Autodesk Inventor part; units mm, degrees
(part 3 of 3)
  arc A48 (19.7098, 5.9019) -> (19.4526, 6.1717) centre (13.25, 0) ccw
  line L1883 (19.7098, 5.9019) -> (19.6582, 5.7672)
  line L1884 (19.6582, 5.7672) -> (19.6285, 5.6961)
  line L1885 (19.6285, 5.6961) -> (19.5685, 5.5641)
  line L1886 (19.5685, 5.5641) -> (19.5095, 5.4477)
  line L1887 (19.5095, 5.4477) -> (19.4525, 5.3459)
  line L1888 (19.4525, 5.3459) -> (19.3981, 5.2575)
  line L1889 (19.3981, 5.2575) -> (19.348, 5.1833)
  line L1890 (19.348, 5.1833) -> (19.3013, 5.1201)
  line L1891 (19.3013, 5.1201) -> (19.2635, 5.0732)
  line L1892 (19.2635, 5.0732) -> (19.2071, 5.0072)
  line L1893 (19.2071, 5.0072) -> (19.1891, 4.9822)
  line L1894 (19.1891, 4.9822) -> (19.1747, 4.9588)
  line L1895 (19.1747, 4.9588) -> (19.1639, 4.937)
  line L1896 (19.1639, 4.937) -> (19.1565, 4.917)
  line L1897 (19.1565, 4.917) -> (19.1525, 4.8989)
  line L1898 (19.1525, 4.8989) -> (19.1519, 4.8829)
  line L1899 (19.1519, 4.8829) -> (19.1544, 4.869)
  line L1900 (19.1544, 4.869) -> (19.1601, 4.8575)
  line L1901 (19.1601, 4.8575) -> (19.1753, 4.8388)
  line L1902 (19.1753, 4.8388) -> (19.2633, 4.7289)
  line L1903 (19.2633, 4.7289) -> (19.3493, 4.6175)
  line L1904 (19.3493, 4.6175) -> (19.3639, 4.5983)
  line L1905 (19.3639, 4.5983) -> (19.3738, 4.5901)
  line L1906 (19.3738, 4.5901) -> (19.3867, 4.5843)
  line L1907 (19.3867, 4.5843) -> (19.4024, 4.5812)
  line L1908 (19.4024, 4.5812) -> (19.4209, 4.5808)
  line L1909 (19.4209, 4.5808) -> (19.4421, 4.5832)
  line L1910 (19.4421, 4.5832) -> (19.4658, 4.5886)
  line L1911 (19.4658, 4.5886) -> (19.492, 4.5971)
  line L1912 (19.492, 4.5971) -> (19.5205, 4.6087)
  line L1913 (19.5205, 4.6087) -> (19.5979, 4.6479)
  line L1914 (19.5979, 4.6479) -> (19.6525, 4.6736)
  line L1915 (19.6525, 4.6736) -> (19.7249, 4.7041)
  line L1916 (19.7249, 4.7041) -> (19.8088, 4.7352)
  line L1917 (19.8088, 4.7352) -> (19.9076, 4.7673)
  line L1918 (19.9076, 4.7673) -> (20.0198, 4.7987)
  line L1919 (20.0198, 4.7987) -> (20.1469, 4.8286)
  line L1920 (20.1469, 4.8286) -> (20.2894, 4.8558)
  line L1921 (20.2894, 4.8558) -> (20.3654, 4.8679)
  line L1922 (20.3654, 4.8679) -> (20.5085, 4.8863)
  arc A49 (20.7101, 4.5727) -> (20.5085, 4.8863) centre (13.25, 0) ccw
  line L1923 (20.7101, 4.5727) -> (20.6338, 4.4502)
  line L1924 (20.6338, 4.4502) -> (20.5912, 4.3861)
  line L1925 (20.5912, 4.3861) -> (20.5073, 4.2678)
  line L1926 (20.5073, 4.2678) -> (20.4273, 4.1646)
  line L1927 (20.4273, 4.1646) -> (20.3522, 4.0755)
  line L1928 (20.3522, 4.0755) -> (20.2819, 3.999)
  line L1929 (20.2819, 3.999) -> (20.2187, 3.9356)
  line L1930 (20.2187, 3.9356) -> (20.1609, 3.8824)
  line L1931 (20.1609, 3.8824) -> (20.1149, 3.8434)
  line L1932 (20.1149, 3.8434) -> (20.0471, 3.7893)
  line L1933 (20.0471, 3.7893) -> (20.0247, 3.7682)
  line L1934 (20.0247, 3.7682) -> (20.0061, 3.7479)
  line L1935 (20.0061, 3.7479) -> (19.9914, 3.7286)
  line L1936 (19.9914, 3.7286) -> (19.9803, 3.7103)
  line L1937 (19.9803, 3.7103) -> (19.973, 3.6933)
  line L1938 (19.973, 3.6933) -> (19.9693, 3.6777)
  line L1939 (19.9693, 3.6777) -> (19.9692, 3.6636)
  line L1940 (19.9692, 3.6636) -> (19.9726, 3.6512)
  line L1941 (19.9726, 3.6512) -> (19.9839, 3.63)
  line L1942 (19.9839, 3.63) -> (20.0496, 3.5054)
  line L1943 (20.0496, 3.5054) -> (20.113, 3.3797)
  line L1944 (20.113, 3.3797) -> (20.1237, 3.3581)
  line L1945 (20.1237, 3.3581) -> (20.1318, 3.3482)
  line L1946 (20.1318, 3.3482) -> (20.1434, 3.3401)
  line L1947 (20.1434, 3.3401) -> (20.1582, 3.3341)
  line L1948 (20.1582, 3.3341) -> (20.1763, 3.3302)
  line L1949 (20.1763, 3.3302) -> (20.1976, 3.3286)
  line L1950 (20.1976, 3.3286) -> (20.2219, 3.3294)
  line L1951 (20.2219, 3.3294) -> (20.2492, 3.3327)
  line L1952 (20.2492, 3.3327) -> (20.2794, 3.3387)
  line L1953 (20.2794, 3.3387) -> (20.3628, 3.3626)
  line L1954 (20.3628, 3.3626) -> (20.4212, 3.3775)
  line L1955 (20.4212, 3.3775) -> (20.4981, 3.3937)
  line L1956 (20.4981, 3.3937) -> (20.5864, 3.4084)
  line L1957 (20.5864, 3.4084) -> (20.6895, 3.4212)
  line L1958 (20.6895, 3.4212) -> (20.8057, 3.4308)
  line L1959 (20.8057, 3.4308) -> (20.9361, 3.4361)
  line L1960 (20.9361, 3.4361) -> (21.0811, 3.4358)
  line L1961 (21.0811, 3.4358) -> (21.1581, 3.4333)
  line L1962 (21.1581, 3.4333) -> (21.3021, 3.4243)
  arc A50 (21.4406, 3.0783) -> (21.3021, 3.4243) centre (13.25, 0) ccw
  line L1963 (21.4406, 3.0783) -> (21.3426, 2.9724)
  line L1964 (21.3426, 2.9724) -> (21.2886, 2.9175)
  line L1965 (21.2886, 2.9175) -> (21.1838, 2.8172)
  line L1966 (21.1838, 2.8172) -> (21.0858, 2.731)
  line L1967 (21.0858, 2.731) -> (20.9951, 2.6578)
  line L1968 (20.9951, 2.6578) -> (20.9117, 2.5959)
  line L1969 (20.9117, 2.5959) -> (20.8376, 2.5457)
  line L1970 (20.8376, 2.5457) -> (20.7708, 2.5043)
  line L1971 (20.7708, 2.5043) -> (20.7182, 2.4748)
  line L1972 (20.7182, 2.4748) -> (20.6414, 2.4345)
  line L1973 (20.6414, 2.4345) -> (20.6154, 2.418)
  line L1974 (20.6154, 2.418) -> (20.5933, 2.4016)
  line L1975 (20.5933, 2.4016) -> (20.5752, 2.3854)
  line L1976 (20.5752, 2.3854) -> (20.5609, 2.3696)
  line L1977 (20.5609, 2.3696) -> (20.5505, 2.3542)
  line L1978 (20.5505, 2.3542) -> (20.5439, 2.3396)
  line L1979 (20.5439, 2.3396) -> (20.5411, 2.3258)
  line L1980 (20.5411, 2.3258) -> (20.5421, 2.313)
  line L1981 (20.5421, 2.313) -> (20.5492, 2.29)
  line L1982 (20.5492, 2.29) -> (20.5901, 2.1553)
  line L1983 (20.5901, 2.1553) -> (20.6286, 2.0198)
  line L1984 (20.6286, 2.0198) -> (20.635, 1.9966)
  line L1985 (20.635, 1.9966) -> (20.6411, 1.9853)
  line L1986 (20.6411, 1.9853) -> (20.6509, 1.9752)
  line L1987 (20.6509, 1.9752) -> (20.6644, 1.9664)
  line L1988 (20.6644, 1.9664) -> (20.6814, 1.9592)
  line L1989 (20.6814, 1.9592) -> (20.702, 1.9536)
  line L1990 (20.702, 1.9536) -> (20.726, 1.9498)
  line L1991 (20.726, 1.9498) -> (20.7534, 1.9479)
  line L1992 (20.7534, 1.9479) -> (20.7842, 1.9481)
  line L1993 (20.7842, 1.9481) -> (20.8706, 1.9557)
  line L1994 (20.8706, 1.9557) -> (20.9308, 1.9593)
  line L1995 (20.9308, 1.9593) -> (21.0094, 1.9606)
  line L1996 (21.0094, 1.9606) -> (21.0989, 1.9584)
  line L1997 (21.0989, 1.9584) -> (21.2025, 1.9515)
  line L1998 (21.2025, 1.9515) -> (21.3184, 1.9389)
  line L1999 (21.3184, 1.9389) -> (21.4474, 1.9194)
  line L2000 (21.4474, 1.9194) -> (21.5898, 1.8917)
  line L2001 (21.5898, 1.8917) -> (21.6649, 1.8746)
  line L2002 (21.6649, 1.8746) -> (21.8047, 1.8386)
  arc A51 (21.8752, 1.4726) -> (21.8047, 1.8386) centre (13.25, 0) ccw
  line L2003 (21.8752, 1.4726) -> (21.7589, 1.3872)
  line L2004 (21.7589, 1.3872) -> (21.6955, 1.3434)
  line L2005 (21.6955, 1.3434) -> (21.5736, 1.2648)
  line L2006 (21.5736, 1.2648) -> (21.461, 1.1987)
  line L2007 (21.461, 1.1987) -> (21.3581, 1.1439)
  line L2008 (21.3581, 1.1439) -> (21.2645, 1.099)
  line L2009 (21.2645, 1.099) -> (21.1823, 1.0637)
  line L2010 (21.1823, 1.0637) -> (21.1088, 1.0358)
  line L2011 (21.1088, 1.0358) -> (21.0516, 1.0167)
  line L2012 (21.0516, 1.0167) -> (20.9685, 0.9916)
  line L2013 (20.9685, 0.9916) -> (20.9399, 0.9804)
  line L2014 (20.9399, 0.9804) -> (20.9151, 0.9685)
  line L2015 (20.9151, 0.9685) -> (20.8942, 0.956)
  line L2016 (20.8942, 0.956) -> (20.8772, 0.9431)
  line L2017 (20.8772, 0.9431) -> (20.8641, 0.9301)
  line L2018 (20.8641, 0.9301) -> (20.8549, 0.917)
  line L2019 (20.8549, 0.917) -> (20.8495, 0.9039)
  line L2020 (20.8495, 0.9039) -> (20.848, 0.8912)
  line L2021 (20.848, 0.8912) -> (20.8507, 0.8672)
  line L2022 (20.8507, 0.8672) -> (20.8654, 0.7272)
  line L2023 (20.8654, 0.7272) -> (20.8775, 0.5869)
  line L2024 (20.8775, 0.5869) -> (20.8794, 0.5629)
  line L2025 (20.8794, 0.5629) -> (20.8833, 0.5506)
  line L2026 (20.8833, 0.5506) -> (20.891, 0.5389)
  line L2027 (20.891, 0.5389) -> (20.9025, 0.5277)
  line L2028 (20.9025, 0.5277) -> (20.9179, 0.5174)
  line L2029 (20.9179, 0.5174) -> (20.937, 0.508)
  line L2030 (20.937, 0.508) -> (20.9599, 0.4997)
  line L2031 (20.9599, 0.4997) -> (20.9865, 0.4926)
  line L2032 (20.9865, 0.4926) -> (21.0167, 0.487)
  line L2033 (21.0167, 0.487) -> (21.103, 0.4781)
  line L2034 (21.103, 0.4781) -> (21.1628, 0.4702)
  line L2035 (21.1628, 0.4702) -> (21.2402, 0.4567)
  line L2036 (21.2402, 0.4567) -> (21.3277, 0.4376)
  line L2037 (21.3277, 0.4376) -> (21.4281, 0.4112)
  line L2038 (21.4281, 0.4112) -> (21.5395, 0.3769)
  line L2039 (21.5395, 0.3769) -> (21.6626, 0.3333)
  line L2040 (21.6626, 0.3333) -> (21.7971, 0.2792)
  line L2041 (21.7971, 0.2792) -> (21.8676, 0.2482)
  line L2042 (21.8676, 0.2482) -> (21.998, 0.1864)
  arc A52 (21.998, -0.1864) -> (21.998, 0.1864) centre (13.25, 0) ccw
  line L2043 (21.998, -0.1864) -> (21.8676, -0.2482)
  line L2044 (21.8676, -0.2482) -> (21.7971, -0.2792)
  line L2045 (21.7971, -0.2792) -> (21.6626, -0.3333)
  line L2046 (21.6626, -0.3333) -> (21.5395, -0.3769)
  line L2047 (21.5395, -0.3769) -> (21.4281, -0.4112)
  line L2048 (21.4281, -0.4112) -> (21.3277, -0.4376)
  line L2049 (21.3277, -0.4376) -> (21.2402, -0.4567)
  line L2050 (21.2402, -0.4567) -> (21.1628, -0.4702)
  line L2051 (21.1628, -0.4702) -> (21.103, -0.4781)
  line L2052 (21.103, -0.4781) -> (21.0167, -0.487)
  line L2053 (21.0167, -0.487) -> (20.9865, -0.4926)
  line L2054 (20.9865, -0.4926) -> (20.9599, -0.4997)
  line L2055 (20.9599, -0.4997) -> (20.937, -0.508)
  line L2056 (20.937, -0.508) -> (20.9179, -0.5174)
  line L2057 (20.9179, -0.5174) -> (20.9025, -0.5277)
  line L2058 (20.9025, -0.5277) -> (20.891, -0.5389)
  line L2059 (20.891, -0.5389) -> (20.8833, -0.5506)
  line L2060 (20.8833, -0.5506) -> (20.8794, -0.5629)
  line L2061 (20.8794, -0.5629) -> (20.8775, -0.5869)
  line L2062 (20.8775, -0.5869) -> (20.8654, -0.7272)
  line L2063 (20.8654, -0.7272) -> (20.8507, -0.8672)
  line L2064 (20.8507, -0.8672) -> (20.848, -0.8912)
  line L2065 (20.848, -0.8912) -> (20.8495, -0.9039)
  line L2066 (20.8495, -0.9039) -> (20.8549, -0.917)
  line L2067 (20.8549, -0.917) -> (20.8641, -0.9301)
  line L2068 (20.8641, -0.9301) -> (20.8772, -0.9431)
  line L2069 (20.8772, -0.9431) -> (20.8942, -0.956)
  line L2070 (20.8942, -0.956) -> (20.9151, -0.9685)
  line L2071 (20.9151, -0.9685) -> (20.9399, -0.9804)
  line L2072 (20.9399, -0.9804) -> (20.9685, -0.9916)
  line L2073 (20.9685, -0.9916) -> (21.0516, -1.0167)
  line L2074 (21.0516, -1.0167) -> (21.1088, -1.0358)
  line L2075 (21.1088, -1.0358) -> (21.1823, -1.0637)
  line L2076 (21.1823, -1.0637) -> (21.2645, -1.099)
  line L2077 (21.2645, -1.099) -> (21.3581, -1.1439)
  line L2078 (21.3581, -1.1439) -> (21.461, -1.1987)
  line L2079 (21.461, -1.1987) -> (21.5736, -1.2648)
  line L2080 (21.5736, -1.2648) -> (21.6955, -1.3434)
  line L2081 (21.6955, -1.3434) -> (21.7589, -1.3872)
  line L2082 (21.7589, -1.3872) -> (21.8752, -1.4726)
  arc A53 (21.8047, -1.8386) -> (21.8752, -1.4726) centre (13.25, 0) ccw
  line L2083 (21.8047, -1.8386) -> (21.6649, -1.8746)
  line L2084 (21.6649, -1.8746) -> (21.5898, -1.8917)
  line L2085 (21.5898, -1.8917) -> (21.4474, -1.9194)
  line L2086 (21.4474, -1.9194) -> (21.3184, -1.9389)
  line L2087 (21.3184, -1.9389) -> (21.2025, -1.9515)
  line L2088 (21.2025, -1.9515) -> (21.0989, -1.9584)
  line L2089 (21.0989, -1.9584) -> (21.0094, -1.9606)
  line L2090 (21.0094, -1.9606) -> (20.9308, -1.9593)
  line L2091 (20.9308, -1.9593) -> (20.8706, -1.9557)
  line L2092 (20.8706, -1.9557) -> (20.7842, -1.9481)
  line L2093 (20.7842, -1.9481) -> (20.7534, -1.9479)
  line L2094 (20.7534, -1.9479) -> (20.726, -1.9498)
  line L2095 (20.726, -1.9498) -> (20.702, -1.9536)
  line L2096 (20.702, -1.9536) -> (20.6814, -1.9592)
  line L2097 (20.6814, -1.9592) -> (20.6644, -1.9664)
  line L2098 (20.6644, -1.9664) -> (20.6509, -1.9752)
  line L2099 (20.6509, -1.9752) -> (20.6411, -1.9853)
  line L2100 (20.6411, -1.9853) -> (20.635, -1.9966)
  line L2101 (20.635, -1.9966) -> (20.6286, -2.0198)
  line L2102 (20.6286, -2.0198) -> (20.5901, -2.1553)
  line L2103 (20.5901, -2.1553) -> (20.5492, -2.29)
  line L2104 (20.5492, -2.29) -> (20.5421, -2.313)
  line L2105 (20.5421, -2.313) -> (20.5411, -2.3258)
  line L2106 (20.5411, -2.3258) -> (20.5439, -2.3396)
  line L2107 (20.5439, -2.3396) -> (20.5505, -2.3542)
  line L2108 (20.5505, -2.3542) -> (20.5609, -2.3696)
  line L2109 (20.5609, -2.3696) -> (20.5752, -2.3854)
  line L2110 (20.5752, -2.3854) -> (20.5933, -2.4016)
  line L2111 (20.5933, -2.4016) -> (20.6154, -2.418)
  line L2112 (20.6154, -2.418) -> (20.6414, -2.4345)
  line L2113 (20.6414, -2.4345) -> (20.7182, -2.4748)
  line L2114 (20.7182, -2.4748) -> (20.7708, -2.5043)
  line L2115 (20.7708, -2.5043) -> (20.8376, -2.5457)
  line L2116 (20.8376, -2.5457) -> (20.9117, -2.5959)
  line L2117 (20.9117, -2.5959) -> (20.9951, -2.6578)
  line L2118 (20.9951, -2.6578) -> (21.0858, -2.731)
  line L2119 (21.0858, -2.731) -> (21.1838, -2.8172)
  line L2120 (21.1838, -2.8172) -> (21.2886, -2.9175)
  line L2121 (21.2886, -2.9175) -> (21.3426, -2.9724)
  line L2122 (21.3426, -2.9724) -> (21.4406, -3.0783)
  arc A54 (21.3021, -3.4243) -> (21.4406, -3.0783) centre (13.25, 0) ccw
  line L2123 (21.3021, -3.4243) -> (21.1581, -3.4333)
  line L2124 (21.1581, -3.4333) -> (21.0811, -3.4358)
  line L2125 (21.0811, -3.4358) -> (20.9361, -3.4361)
  line L2126 (20.9361, -3.4361) -> (20.8057, -3.4308)
  line L2127 (20.8057, -3.4308) -> (20.6895, -3.4212)
  line L2128 (20.6895, -3.4212) -> (20.5864, -3.4084)
  line L2129 (20.5864, -3.4084) -> (20.4981, -3.3937)
  line L2130 (20.4981, -3.3937) -> (20.4212, -3.3775)
  line L2131 (20.4212, -3.3775) -> (20.3628, -3.3626)
  line L2132 (20.3628, -3.3626) -> (20.2794, -3.3387)
  line L2133 (20.2794, -3.3387) -> (20.2492, -3.3327)
  line L2134 (20.2492, -3.3327) -> (20.2219, -3.3294)
  line L2135 (20.2219, -3.3294) -> (20.1976, -3.3286)
  line L2136 (20.1976, -3.3286) -> (20.1763, -3.3302)
  line L2137 (20.1763, -3.3302) -> (20.1582, -3.3341)
  line L2138 (20.1582, -3.3341) -> (20.1434, -3.3401)
  line L2139 (20.1434, -3.3401) -> (20.1318, -3.3482)
  line L2140 (20.1318, -3.3482) -> (20.1237, -3.3581)
  line L2141 (20.1237, -3.3581) -> (20.113, -3.3797)
  line L2142 (20.113, -3.3797) -> (20.0496, -3.5054)
  line L2143 (20.0496, -3.5054) -> (19.9839, -3.63)
  line L2144 (19.9839, -3.63) -> (19.9726, -3.6512)
  line L2145 (19.9726, -3.6512) -> (19.9692, -3.6636)
  line L2146 (19.9692, -3.6636) -> (19.9693, -3.6777)
  line L2147 (19.9693, -3.6777) -> (19.973, -3.6933)
  line L2148 (19.973, -3.6933) -> (19.9803, -3.7103)
  line L2149 (19.9803, -3.7103) -> (19.9914, -3.7286)
  line L2150 (19.9914, -3.7286) -> (20.0061, -3.7479)
  line L2151 (20.0061, -3.7479) -> (20.0247, -3.7682)
  line L2152 (20.0247, -3.7682) -> (20.0471, -3.7893)
  line L2153 (20.0471, -3.7893) -> (20.1149, -3.8434)
  line L2154 (20.1149, -3.8434) -> (20.1609, -3.8824)
  line L2155 (20.1609, -3.8824) -> (20.2187, -3.9356)
  line L2156 (20.2187, -3.9356) -> (20.2819, -3.999)
  line L2157 (20.2819, -3.999) -> (20.3522, -4.0755)
  line L2158 (20.3522, -4.0755) -> (20.4273, -4.1646)
  line L2159 (20.4273, -4.1646) -> (20.5073, -4.2678)
  line L2160 (20.5073, -4.2678) -> (20.5912, -4.3861)
  line L2161 (20.5912, -4.3861) -> (20.6338, -4.4502)
  line L2162 (20.6338, -4.4502) -> (20.7101, -4.5727)
  arc A55 (20.5085, -4.8863) -> (20.7101, -4.5727) centre (13.25, 0) ccw
  line L2163 (20.5085, -4.8863) -> (20.3654, -4.8679)
  line L2164 (20.3654, -4.8679) -> (20.2894, -4.8558)
  line L2165 (20.2894, -4.8558) -> (20.1469, -4.8286)
  line L2166 (20.1469, -4.8286) -> (20.0198, -4.7987)
  line L2167 (20.0198, -4.7987) -> (19.9076, -4.7673)
  line L2168 (19.9076, -4.7673) -> (19.8088, -4.7352)
  line L2169 (19.8088, -4.7352) -> (19.7249, -4.7041)
  line L2170 (19.7249, -4.7041) -> (19.6525, -4.6736)
  line L2171 (19.6525, -4.6736) -> (19.5979, -4.6479)
  line L2172 (19.5979, -4.6479) -> (19.5205, -4.6087)
  line L2173 (19.5205, -4.6087) -> (19.492, -4.5971)
  line L2174 (19.492, -4.5971) -> (19.4658, -4.5886)
  line L2175 (19.4658, -4.5886) -> (19.4421, -4.5832)
  line L2176 (19.4421, -4.5832) -> (19.4209, -4.5808)
  line L2177 (19.4209, -4.5808) -> (19.4024, -4.5812)
  line L2178 (19.4024, -4.5812) -> (19.3867, -4.5843)
  line L2179 (19.3867, -4.5843) -> (19.3738, -4.5901)
  line L2180 (19.3738, -4.5901) -> (19.3639, -4.5983)
  line L2181 (19.3639, -4.5983) -> (19.3493, -4.6175)
  line L2182 (19.3493, -4.6175) -> (19.2633, -4.7289)
  line L2183 (19.2633, -4.7289) -> (19.1753, -4.8388)
  line L2184 (19.1753, -4.8388) -> (19.1601, -4.8575)
  line L2185 (19.1601, -4.8575) -> (19.1544, -4.869)
  line L2186 (19.1544, -4.869) -> (19.1519, -4.8829)
  line L2187 (19.1519, -4.8829) -> (19.1525, -4.8989)
  line L2188 (19.1525, -4.8989) -> (19.1565, -4.917)
  line L2189 (19.1565, -4.917) -> (19.1639, -4.937)
  line L2190 (19.1639, -4.937) -> (19.1747, -4.9588)
  line L2191 (19.1747, -4.9588) -> (19.1891, -4.9822)
  line L2192 (19.1891, -4.9822) -> (19.2071, -5.0072)
  line L2193 (19.2071, -5.0072) -> (19.2635, -5.0732)
  line L2194 (19.2635, -5.0732) -> (19.3013, -5.1201)
  line L2195 (19.3013, -5.1201) -> (19.348, -5.1833)
  line L2196 (19.348, -5.1833) -> (19.3981, -5.2575)
  line L2197 (19.3981, -5.2575) -> (19.4525, -5.3459)
  line L2198 (19.4525, -5.3459) -> (19.5095, -5.4477)
  line L2199 (19.5095, -5.4477) -> (19.5685, -5.5641)
  line L2200 (19.5685, -5.5641) -> (19.6285, -5.6961)
  line L2201 (19.6285, -5.6961) -> (19.6582, -5.7672)
  line L2202 (19.6582, -5.7672) -> (19.7098, -5.9019)
  arc A56 (19.4526, -6.1717) -> (19.7098, -5.9019) centre (13.25, 0) ccw
  line L2203 (19.4526, -6.1717) -> (19.3156, -6.1265)
  line L2204 (19.3156, -6.1265) -> (19.2432, -6.1002)
  line L2205 (19.2432, -6.1002) -> (19.1084, -6.0465)
  line L2206 (19.1084, -6.0465) -> (18.9893, -5.9932)
  line L2207 (18.9893, -5.9932) -> (18.885, -5.9411)
  line L2208 (18.885, -5.9411) -> (18.7941, -5.8909)
  line L2209 (18.7941, -5.8909) -> (18.7176, -5.8444)
  line L2210 (18.7176, -5.8444) -> (18.6523, -5.8008)
  line L2211 (18.6523, -5.8008) -> (18.6036, -5.7653)
  line L2212 (18.6036, -5.7653) -> (18.5349, -5.7121)
  line L2213 (18.5349, -5.7121) -> (18.5092, -5.6953)
  line L2214 (18.5092, -5.6953) -> (18.4851, -5.6821)
  line L2215 (18.4851, -5.6821) -> (18.4628, -5.6723)
  line L2216 (18.4628, -5.6723) -> (18.4425, -5.6659)
  line L2217 (18.4425, -5.6659) -> (18.4242, -5.6628)
  line L2218 (18.4242, -5.6628) -> (18.4082, -5.6629)
  line L2219 (18.4082, -5.6629) -> (18.3945, -5.6661)
  line L2220 (18.3945, -5.6661) -> (18.3832, -5.6723)
  line L2221 (18.3832, -5.6723) -> (18.3653, -5.6883)
  line L2222 (18.3653, -5.6883) -> (18.2597, -5.7815)
  line L2223 (18.2597, -5.7815) -> (18.1524, -5.8727)
  line L2224 (18.1524, -5.8727) -> (18.134, -5.8882)
  line L2225 (18.134, -5.8882) -> (18.1262, -5.8985)
  line L2226 (18.1262, -5.8985) -> (18.1211, -5.9116)
  line L2227 (18.1211, -5.9116) -> (18.1188, -5.9275)
  line L2228 (18.1188, -5.9275) -> (18.1192, -5.946)
  line L2229 (18.1192, -5.946) -> (18.1227, -5.967)
  line L2230 (18.1227, -5.967) -> (18.1292, -5.9904)
  line L2231 (18.1292, -5.9904) -> (18.1389, -6.0162)
  line L2232 (18.1389, -6.0162) -> (18.1518, -6.0441)
  line L2233 (18.1518, -6.0441) -> (18.1947, -6.1196)
  line L2234 (18.1947, -6.1196) -> (18.2229, -6.1728)
  line L2235 (18.2229, -6.1728) -> (18.2568, -6.2437)
  line L2236 (18.2568, -6.2437) -> (18.292, -6.326)
  line L2237 (18.292, -6.326) -> (18.3287, -6.4232)
  line L2238 (18.3287, -6.4232) -> (18.3654, -6.5338)
  line L2239 (18.3654, -6.5338) -> (18.4013, -6.6593)
  line L2240 (18.4013, -6.6593) -> (18.4352, -6.8003)
  line L2241 (18.4352, -6.8003) -> (18.4509, -6.8757)
  line L2242 (18.4509, -6.8757) -> (18.4762, -7.0178)
  arc A57 (18.1725, -7.234) -> (18.4762, -7.0178) centre (13.25, 0) ccw
  line L2243 (18.1725, -7.234) -> (18.0465, -7.1637)
  line L2244 (18.0465, -7.1637) -> (17.9804, -7.1242)
  line L2245 (17.9804, -7.1242) -> (17.8583, -7.046)
  line L2246 (17.8583, -7.046) -> (17.7514, -6.9711)
  line L2247 (17.7514, -6.9711) -> (17.6588, -6.9002)
  line L2248 (17.6588, -6.9002) -> (17.5791, -6.8337)
  line L2249 (17.5791, -6.8337) -> (17.5128, -6.7736)
  line L2250 (17.5128, -6.7736) -> (17.4568, -6.7184)
  line L2251 (17.4568, -6.7184) -> (17.4157, -6.6742)
  line L2252 (17.4157, -6.6742) -> (17.3584, -6.6091)
  line L2253 (17.3584, -6.6091) -> (17.3363, -6.5877)
  line L2254 (17.3363, -6.5877) -> (17.3151, -6.5701)
  line L2255 (17.3151, -6.5701) -> (17.2951, -6.5563)
  line L2256 (17.2951, -6.5563) -> (17.2764, -6.5462)
  line L2257 (17.2764, -6.5462) -> (17.259, -6.5397)
  line L2258 (17.259, -6.5397) -> (17.2433, -6.5367)
  line L2259 (17.2433, -6.5367) -> (17.2292, -6.5373)
  line L2260 (17.2292, -6.5373) -> (17.217, -6.5412)
  line L2261 (17.217, -6.5412) -> (17.1963, -6.5536)
  line L2262 (17.1963, -6.5536) -> (17.075, -6.6251)
  line L2263 (17.075, -6.6251) -> (16.9524, -6.6944)
  line L2264 (16.9524, -6.6944) -> (16.9314, -6.7061)
  line L2265 (16.9314, -6.7061) -> (16.9218, -6.7147)
  line L2266 (16.9218, -6.7147) -> (16.9143, -6.7266)
  line L2267 (16.9143, -6.7266) -> (16.909, -6.7418)
  line L2268 (16.909, -6.7418) -> (16.906, -6.76)
  line L2269 (16.906, -6.76) -> (16.9054, -6.7813)
  line L2270 (16.9054, -6.7813) -> (16.9073, -6.8056)
  line L2271 (16.9073, -6.8056) -> (16.912, -6.8327)
  line L2272 (16.912, -6.8327) -> (16.9194, -6.8625)
  line L2273 (16.9194, -6.8625) -> (16.9472, -6.9448)
  line L2274 (16.9472, -6.9448) -> (16.9649, -7.0024)
  line L2275 (16.9649, -7.0024) -> (16.9847, -7.0784)
  line L2276 (16.9847, -7.0784) -> (17.0036, -7.1659)
  line L2277 (17.0036, -7.1659) -> (17.0214, -7.2683)
  line L2278 (17.0214, -7.2683) -> (17.0364, -7.3838)
  line L2279 (17.0364, -7.3838) -> (17.0479, -7.5139)
  line L2280 (17.0479, -7.5139) -> (17.0545, -7.6588)
  line L2281 (17.0545, -7.6588) -> (17.0557, -7.7357)
  line L2282 (17.0557, -7.7357) -> (17.0536, -7.88)
  arc A58 (16.7145, -8.0349) -> (17.0536, -7.88) centre (13.25, 0) ccw
  line L2283 (16.7145, -8.0349) -> (16.6041, -7.942)
  line L2284 (16.6041, -7.942) -> (16.5467, -7.8907)
  line L2285 (16.5467, -7.8907) -> (16.4415, -7.7908)
  line L2286 (16.4415, -7.7908) -> (16.3508, -7.697)
  line L2287 (16.3508, -7.697) -> (16.2733, -7.6099)
  line L2288 (16.2733, -7.6099) -> (16.2075, -7.5295)
  line L2289 (16.2075, -7.5295) -> (16.1538, -7.4579)
  line L2290 (16.1538, -7.4579) -> (16.1094, -7.3931)
  line L2291 (16.1094, -7.3931) -> (16.0773, -7.342)
  line L2292 (16.0773, -7.342) -> (16.0334, -7.2672)
  line L2293 (16.0334, -7.2672) -> (16.0157, -7.242)
  line L2294 (16.0157, -7.242) -> (15.9983, -7.2207)
  line L2295 (15.9983, -7.2207) -> (15.9812, -7.2034)
  line L2296 (15.9812, -7.2034) -> (15.9647, -7.1899)
  line L2297 (15.9647, -7.1899) -> (15.949, -7.1802)
  line L2298 (15.949, -7.1802) -> (15.934, -7.1743)
  line L2299 (15.934, -7.1743) -> (15.9201, -7.1722)
  line L2300 (15.9201, -7.1722) -> (15.9073, -7.1738)
  line L2301 (15.9073, -7.1738) -> (15.8847, -7.182)
  line L2302 (15.8847, -7.182) -> (15.7521, -7.2293)
  line L2303 (15.7521, -7.2293) -> (15.6186, -7.2741)
  line L2304 (15.6186, -7.2741) -> (15.5957, -7.2816)
  line L2305 (15.5957, -7.2816) -> (15.5847, -7.2883)
  line L2306 (15.5847, -7.2883) -> (15.5751, -7.2986)
  line L2307 (15.5751, -7.2986) -> (15.567, -7.3124)
  line L2308 (15.567, -7.3124) -> (15.5605, -7.3298)
  line L2309 (15.5605, -7.3298) -> (15.5559, -7.3506)
  line L2310 (15.5559, -7.3506) -> (15.5533, -7.3747)
  line L2311 (15.5533, -7.3747) -> (15.5527, -7.4022)
  line L2312 (15.5527, -7.4022) -> (15.5544, -7.433)
  line L2313 (15.5544, -7.433) -> (15.5661, -7.519)
  line L2314 (15.5661, -7.519) -> (15.5725, -7.5789)
  line L2315 (15.5725, -7.5789) -> (15.5776, -7.6573)
  line L2316 (15.5776, -7.6573) -> (15.5796, -7.7468)
  line L2317 (15.5796, -7.7468) -> (15.5777, -7.8506)
  line L2318 (15.5777, -7.8506) -> (15.5706, -7.967)
  line L2319 (15.5706, -7.967) -> (15.5572, -8.0968)
  line L2320 (15.5572, -8.0968) -> (15.5364, -8.2404)
  line L2321 (15.5364, -8.2404) -> (15.5229, -8.3162)
  line L2322 (15.5229, -8.3162) -> (15.4935, -8.4575)
  arc A59 (15.1313, -8.5454) -> (15.4935, -8.4575) centre (13.25, 0) ccw
  line L2323 (15.1313, -8.5454) -> (15.0404, -8.4332)
  line L2324 (15.0404, -8.4332) -> (14.9938, -8.372)
  line L2325 (14.9938, -8.372) -> (14.9094, -8.254)
  line L2326 (14.9094, -8.254) -> (14.8381, -8.1447)
  line L2327 (14.8381, -8.1447) -> (14.7785, -8.0445)
  line L2328 (14.7785, -8.0445) -> (14.7291, -7.9531)
  line L2329 (14.7291, -7.9531) -> (14.6899, -7.8727)
  line L2330 (14.6899, -7.8727) -> (14.6585, -7.8006)
  line L2331 (14.6585, -7.8006) -> (14.6368, -7.7444)
  line L2332 (14.6368, -7.7444) -> (14.6078, -7.6626)
  line L2333 (14.6078, -7.6626) -> (14.5952, -7.6345)
  line L2334 (14.5952, -7.6345) -> (14.5821, -7.6104)
  line L2335 (14.5821, -7.6104) -> (14.5686, -7.5901)
  line L2336 (14.5686, -7.5901) -> (14.555, -7.5737)
  line L2337 (14.555, -7.5737) -> (14.5413, -7.5612)
  line L2338 (14.5413, -7.5612) -> (14.5278, -7.5526)
  line L2339 (14.5278, -7.5526) -> (14.5145, -7.5479)
  line L2340 (14.5145, -7.5479) -> (14.5017, -7.547)
  line L2341 (14.5017, -7.547) -> (14.4779, -7.5508)
  line L2342 (14.4779, -7.5508) -> (14.3387, -7.5721)
  line L2343 (14.3387, -7.5721) -> (14.1992, -7.5909)
  line L2344 (14.1992, -7.5909) -> (14.1753, -7.594)
  line L2345 (14.1753, -7.594) -> (14.1632, -7.5984)
  line L2346 (14.1632, -7.5984) -> (14.1518, -7.6067)
  line L2347 (14.1518, -7.6067) -> (14.1412, -7.6187)
  line L2348 (14.1412, -7.6187) -> (14.1316, -7.6346)
  line L2349 (14.1316, -7.6346) -> (14.1232, -7.6541)
  line L2350 (14.1232, -7.6541) -> (14.116, -7.6774)
  line L2351 (14.116, -7.6774) -> (14.1102, -7.7043)
  line L2352 (14.1102, -7.7043) -> (14.106, -7.7347)
  line L2353 (14.106, -7.7347) -> (14.1013, -7.8214)
  line L2354 (14.1013, -7.8214) -> (14.0962, -7.8815)
  line L2355 (14.0962, -7.8815) -> (14.0864, -7.9594)
  line L2356 (14.0864, -7.9594) -> (14.0714, -8.0477)
  line L2357 (14.0714, -8.0477) -> (14.0499, -8.1493)
  line L2358 (14.0499, -8.1493) -> (14.0209, -8.2622)
  line L2359 (14.0209, -8.2622) -> (13.9832, -8.3872)
  line L2360 (13.9832, -8.3872) -> (13.9355, -8.5242)
  line L2361 (13.9355, -8.5242) -> (13.908, -8.5961)
  line L2362 (13.908, -8.5961) -> (13.8524, -8.7292)
  arc A60 (13.4801, -8.747) -> (13.8524, -8.7292) centre (13.25, 0) ccw
  line L2363 (13.4801, -8.747) -> (13.4121, -8.6197)
  line L2364 (13.4121, -8.6197) -> (13.3778, -8.5507)
  line L2365 (13.3778, -8.5507) -> (13.3174, -8.4189)
  line L2366 (13.3174, -8.4189) -> (13.268, -8.2981)
  line L2367 (13.268, -8.2981) -> (13.2284, -8.1884)
  line L2368 (13.2284, -8.1884) -> (13.1973, -8.0893)
  line L2369 (13.1973, -8.0893) -> (13.174, -8.0029)
  line L2370 (13.174, -8.0029) -> (13.1568, -7.9262)
  line L2371 (13.1568, -7.9262) -> (13.1461, -7.8669)
  line L2372 (13.1461, -7.8669) -> (13.1331, -7.7811)
  line L2373 (13.1331, -7.7811) -> (13.126, -7.7511)
  line L2374 (13.126, -7.7511) -> (13.1177, -7.7249)
  line L2375 (13.1177, -7.7249) -> (13.1084, -7.7025)
  line L2376 (13.1084, -7.7025) -> (13.0981, -7.6838)
  line L2377 (13.0981, -7.6838) -> (13.087, -7.669)
  line L2378 (13.087, -7.669) -> (13.0753, -7.658)
  line L2379 (13.0753, -7.658) -> (13.0632, -7.6508)
  line L2380 (13.0632, -7.6508) -> (13.0508, -7.6475)
  line L2381 (13.0508, -7.6475) -> (13.0267, -7.6468)
  line L2382 (13.0267, -7.6468) -> (12.886, -7.6413)
  line L2383 (12.886, -7.6413) -> (12.7454, -7.6334)
  line L2384 (12.7454, -7.6334) -> (12.7214, -7.6318)
  line L2385 (12.7214, -7.6318) -> (12.7087, -7.6339)
  line L2386 (12.7087, -7.6339) -> (12.6959, -7.6399)
  line L2387 (12.6959, -7.6399) -> (12.6833, -7.6497)
  line L2388 (12.6833, -7.6497) -> (12.6708, -7.6635)
  line L2389 (12.6708, -7.6635) -> (12.6588, -7.6811)
  line L2390 (12.6588, -7.6811) -> (12.6474, -7.7025)
  line L2391 (12.6474, -7.7025) -> (12.6366, -7.7278)
  line L2392 (12.6366, -7.7278) -> (12.6267, -7.757)
  line L2393 (12.6267, -7.757) -> (12.6057, -7.8412)
  line L2394 (12.6057, -7.8412) -> (12.5893, -7.8992)
  line L2395 (12.5893, -7.8992) -> (12.5649, -7.9739)
  line L2396 (12.5649, -7.9739) -> (12.5336, -8.0577)
  line L2397 (12.5336, -8.0577) -> (12.4931, -8.1534)
  line L2398 (12.4931, -8.1534) -> (12.4433, -8.2588)
  line L2399 (12.4433, -8.2588) -> (12.3827, -8.3744)
  line L2400 (12.3827, -8.3744) -> (12.3099, -8.4999)
  line L2401 (12.3099, -8.4999) -> (12.2693, -8.5652)
  line L2402 (12.2693, -8.5652) -> (12.1895, -8.6855)
  arc A61 (11.8205, -8.6324) -> (12.1895, -8.6855) centre (13.25, 0) ccw
  line L2403 (11.8205, -8.6324) -> (11.7779, -8.4946)
  line L2404 (11.7779, -8.4946) -> (11.7573, -8.4204)
  line L2405 (11.7573, -8.4204) -> (11.7229, -8.2795)
  line L2406 (11.7229, -8.2795) -> (11.6972, -8.1515)
  line L2407 (11.6972, -8.1515) -> (11.6791, -8.0364)
  line L2408 (11.6791, -8.0364) -> (11.6673, -7.9332)
  line L2409 (11.6673, -7.9332) -> (11.6608, -7.8439)
  line L2410 (11.6608, -7.8439) -> (11.6584, -7.7654)
  line L2411 (11.6584, -7.7654) -> (11.6591, -7.7051)
  line L2412 (11.6591, -7.7051) -> (11.6626, -7.6183)
  line L2413 (11.6626, -7.6183) -> (11.6614, -7.5876)
  line L2414 (11.6614, -7.5876) -> (11.6582, -7.5603)
  line L2415 (11.6582, -7.5603) -> (11.6532, -7.5365)
  line L2416 (11.6532, -7.5365) -> (11.6467, -7.5162)
  line L2417 (11.6467, -7.5162) -> (11.6386, -7.4995)
  line L2418 (11.6386, -7.4995) -> (11.6292, -7.4865)
  line L2419 (11.6292, -7.4865) -> (11.6187, -7.4772)
  line L2420 (11.6187, -7.4772) -> (11.6071, -7.4716)
  line L2421 (11.6071, -7.4716) -> (11.5836, -7.4663)
  line L2422 (11.5836, -7.4663) -> (11.4464, -7.4344)
  line L2423 (11.4464, -7.4344) -> (11.3099, -7.3999)
  line L2424 (11.3099, -7.3999) -> (11.2866, -7.3939)
  line L2425 (11.2866, -7.3939) -> (11.2737, -7.3935)
  line L2426 (11.2737, -7.3935) -> (11.2601, -7.397)
  line L2427 (11.2601, -7.397) -> (11.2458, -7.4042)
  line L2428 (11.2458, -7.4042) -> (11.231, -7.4154)
  line L2429 (11.231, -7.4154) -> (11.2159, -7.4304)
  line L2430 (11.2159, -7.4304) -> (11.2005, -7.4493)
  line L2431 (11.2005, -7.4493) -> (11.1852, -7.4721)
  line L2432 (11.1852, -7.4721) -> (11.17, -7.4988)
  line L2433 (11.17, -7.4988) -> (11.1334, -7.5775)
  line L2434 (11.1334, -7.5775) -> (11.1063, -7.6314)
  line L2435 (11.1063, -7.6314) -> (11.0683, -7.7001)
  line L2436 (11.0683, -7.7001) -> (11.0216, -7.7765)
  line L2437 (11.0216, -7.7765) -> (10.9638, -7.8628)
  line L2438 (10.9638, -7.8628) -> (10.8949, -7.9569)
  line L2439 (10.8949, -7.9569) -> (10.8135, -8.0589)
  line L2440 (10.8135, -8.0589) -> (10.7183, -8.1683)
  line L2441 (10.7183, -8.1683) -> (10.666, -8.2249)
  line L2442 (10.666, -8.2249) -> (10.5649, -8.3278)
  arc A62 (10.2127, -8.2059) -> (10.5649, -8.3278) centre (13.25, 0) ccw
  line L2443 (10.2127, -8.2059) -> (10.1969, -8.0625)
  line L2444 (10.1969, -8.0625) -> (10.1907, -7.9857)
  line L2445 (10.1907, -7.9857) -> (10.1836, -7.8409)
  line L2446 (10.1836, -7.8409) -> (10.1826, -7.7103)
  line L2447 (10.1826, -7.7103) -> (10.1866, -7.5938)
  line L2448 (10.1866, -7.5938) -> (10.1945, -7.4903)
  line L2449 (10.1945, -7.4903) -> (10.2051, -7.4014)
  line L2450 (10.2051, -7.4014) -> (10.2176, -7.3238)
  line L2451 (10.2176, -7.3238) -> (10.2297, -7.2647)
  line L2452 (10.2297, -7.2647) -> (10.2495, -7.1803)
  line L2453 (10.2495, -7.1803) -> (10.2541, -7.1498)
  line L2454 (10.2541, -7.1498) -> (10.2561, -7.1224)
  line L2455 (10.2561, -7.1224) -> (10.2558, -7.0981)
  line L2456 (10.2558, -7.0981) -> (10.2532, -7.0769)
  line L2457 (10.2532, -7.0769) -> (10.2484, -7.059)
  line L2458 (10.2484, -7.059) -> (10.2417, -7.0445)
  line L2459 (10.2417, -7.0445) -> (10.2331, -7.0333)
  line L2460 (10.2331, -7.0333) -> (10.2227, -7.0257)
  line L2461 (10.2227, -7.0257) -> (10.2007, -7.016)
  line L2462 (10.2007, -7.016) -> (10.0721, -6.9587)
  line L2463 (10.0721, -6.9587) -> (9.9445, -6.899)
  line L2464 (9.9445, -6.899) -> (9.9228, -6.8887)
  line L2465 (9.9228, -6.8887) -> (9.9102, -6.8859)
  line L2466 (9.9102, -6.8859) -> (9.8962, -6.8867)
  line L2467 (9.8962, -6.8867) -> (9.8807, -6.8911)
  line L2468 (9.8807, -6.8911) -> (9.8641, -6.8993)
  line L2469 (9.8641, -6.8993) -> (9.8464, -6.9111)
  line L2470 (9.8464, -6.9111) -> (9.8278, -6.9268)
  line L2471 (9.8278, -6.9268) -> (9.8084, -6.9463)
  line L2472 (9.8084, -6.9463) -> (9.7884, -6.9697)
  line L2473 (9.7884, -6.9697) -> (9.7376, -7.04)
  line L2474 (9.7376, -7.04) -> (9.7008, -7.0878)
  line L2475 (9.7008, -7.0878) -> (9.6504, -7.1481)
  line L2476 (9.6504, -7.1481) -> (9.5901, -7.2143)
  line L2477 (9.5901, -7.2143) -> (9.5171, -7.2881)
  line L2478 (9.5171, -7.2881) -> (9.4316, -7.3674)
  line L2479 (9.4316, -7.3674) -> (9.3324, -7.4521)
  line L2480 (9.3324, -7.4521) -> (9.2182, -7.5416)
  line L2481 (9.2182, -7.5416) -> (9.1562, -7.5872)
  line L2482 (9.1562, -7.5872) -> (9.0374, -7.6692)
  arc A63 (8.7146, -7.4828) -> (9.0374, -7.6692) centre (13.25, 0) ccw
  line L2483 (8.7146, -7.4828) -> (8.7262, -7.339)
  line L2484 (8.7262, -7.339) -> (8.7347, -7.2624)
  line L2485 (8.7347, -7.2624) -> (8.7551, -7.1188)
  line L2486 (8.7551, -7.1188) -> (8.7788, -6.9905)
  line L2487 (8.7788, -6.9905) -> (8.8048, -6.8769)
  line L2488 (8.8048, -6.8769) -> (8.8322, -6.7767)
  line L2489 (8.8322, -6.7767) -> (8.8594, -6.6914)
  line L2490 (8.8594, -6.6914) -> (8.8863, -6.6176)
  line L2491 (8.8863, -6.6176) -> (8.9094, -6.5619)
  line L2492 (8.9094, -6.5619) -> (8.9449, -6.4827)
  line L2493 (8.9449, -6.4827) -> (8.9551, -6.4536)
  line L2494 (8.9551, -6.4536) -> (8.9623, -6.4271)
  line L2495 (8.9623, -6.4271) -> (8.9666, -6.4032)
  line L2496 (8.9666, -6.4032) -> (8.968, -6.3819)
  line L2497 (8.968, -6.3819) -> (8.9667, -6.3634)
  line L2498 (8.9667, -6.3634) -> (8.9629, -6.3479)
  line L2499 (8.9629, -6.3479) -> (8.9565, -6.3353)
  line L2500 (8.9565, -6.3353) -> (8.9478, -6.3258)
  line L2501 (8.9478, -6.3258) -> (8.928, -6.3121)
  line L2502 (8.928, -6.3121) -> (8.8126, -6.2315)
  line L2503 (8.8126, -6.2315) -> (8.6986, -6.1488)
  line L2504 (8.6986, -6.1488) -> (8.6792, -6.1345)
  line L2505 (8.6792, -6.1345) -> (8.6674, -6.1294)
  line L2506 (8.6674, -6.1294) -> (8.6535, -6.1275)
  line L2507 (8.6535, -6.1275) -> (8.6375, -6.129)
  line L2508 (8.6375, -6.129) -> (8.6196, -6.1338)
  line L2509 (8.6196, -6.1338) -> (8.6, -6.1421)
  line L2510 (8.6, -6.1421) -> (8.5787, -6.154)
  line L2511 (8.5787, -6.154) -> (8.556, -6.1694)
  line L2512 (8.556, -6.1694) -> (8.532, -6.1886)
  line L2513 (8.532, -6.1886) -> (8.4687, -6.248)
  line L2514 (8.4687, -6.248) -> (8.4236, -6.2881)
  line L2515 (8.4236, -6.2881) -> (8.3627, -6.3377)
  line L2516 (8.3627, -6.3377) -> (8.291, -6.3913)
  line L2517 (8.291, -6.3913) -> (8.2052, -6.4499)
  line L2518 (8.2052, -6.4499) -> (8.1063, -6.5116)
  line L2519 (8.1063, -6.5116) -> (7.9928, -6.576)
  line L2520 (7.9928, -6.576) -> (7.8638, -6.6423)
  line L2521 (7.8638, -6.6423) -> (7.7943, -6.6753)
  line L2522 (7.7943, -6.6753) -> (7.6621, -6.7334)
  arc A64 (7.3804, -6.4893) -> (7.6621, -6.7334) centre (13.25, 0) ccw
  line L2523 (7.3804, -6.4893) -> (7.4191, -6.3502)
  line L2524 (7.4191, -6.3502) -> (7.4418, -6.2767)
  line L2525 (7.4418, -6.2767) -> (7.4891, -6.1395)
  line L2526 (7.4891, -6.1395) -> (7.5367, -6.018)
  line L2527 (7.5367, -6.018) -> (7.5837, -5.9113)
  line L2528 (7.5837, -5.9113) -> (7.6295, -5.8181)
  line L2529 (7.6295, -5.8181) -> (7.6724, -5.7395)
  line L2530 (7.6724, -5.7395) -> (7.7128, -5.6722)
  line L2531 (7.7128, -5.6722) -> (7.746, -5.6218)
  line L2532 (7.746, -5.6218) -> (7.7958, -5.5508)
  line L2533 (7.7958, -5.5508) -> (7.8114, -5.5242)
  line L2534 (7.8114, -5.5242) -> (7.8235, -5.4995)
  line L2535 (7.8235, -5.4995) -> (7.8322, -5.4768)
  line L2536 (7.8322, -5.4768) -> (7.8376, -5.4562)
  line L2537 (7.8376, -5.4562) -> (7.8399, -5.4378)
  line L2538 (7.8399, -5.4378) -> (7.839, -5.4218)
  line L2539 (7.839, -5.4218) -> (7.8352, -5.4082)
  line L2540 (7.8352, -5.4082) -> (7.8284, -5.3973)
  line L2541 (7.8284, -5.3973) -> (7.8115, -5.3801)
  line L2542 (7.8115, -5.3801) -> (7.7134, -5.2791)
  line L2543 (7.7134, -5.2791) -> (7.6172, -5.1763)
  line L2544 (7.6172, -5.1763) -> (7.6008, -5.1586)
  line L2545 (7.6008, -5.1586) -> (7.5902, -5.1514)
  line L2546 (7.5902, -5.1514) -> (7.5769, -5.1469)
  line L2547 (7.5769, -5.1469) -> (7.5609, -5.1453)
  line L2548 (7.5609, -5.1453) -> (7.5424, -5.1466)
  line L2549 (7.5424, -5.1466) -> (7.5216, -5.1511)
  line L2550 (7.5216, -5.1511) -> (7.4985, -5.1587)
  line L2551 (7.4985, -5.1587) -> (7.4733, -5.1696)
  line L2552 (7.4733, -5.1696) -> (7.446, -5.1839)
  line L2553 (7.446, -5.1839) -> (7.3727, -5.2303)
  line L2554 (7.3727, -5.2303) -> (7.3208, -5.261)
  line L2555 (7.3208, -5.261) -> (7.2516, -5.2982)
  line L2556 (7.2516, -5.2982) -> (7.171, -5.3373)
  line L2557 (7.171, -5.3373) -> (7.0758, -5.3786)
  line L2558 (7.0758, -5.3786) -> (6.967, -5.4205)
  line L2559 (6.967, -5.4205) -> (6.8433, -5.4623)
  line L2560 (6.8433, -5.4623) -> (6.7041, -5.5029)
  line L2561 (6.7041, -5.5029) -> (6.6295, -5.5222)
  line L2562 (6.6295, -5.5222) -> (6.4888, -5.5542)
  arc A65 (6.2584, -5.2612) -> (6.4888, -5.5542) centre (13.25, 0) ccw
  line L2563 (6.2584, -5.2612) -> (6.3226, -5.1319)
  line L2564 (6.3226, -5.1319) -> (6.3589, -5.064)
  line L2565 (6.3589, -5.064) -> (6.4313, -4.9383)
  line L2566 (6.4313, -4.9383) -> (6.501, -4.828)
  line L2567 (6.501, -4.828) -> (6.5674, -4.7321)
  line L2568 (6.5674, -4.7321) -> (6.63, -4.6493)
  line L2569 (6.63, -4.6493) -> (6.6869, -4.5802)
  line L2570 (6.6869, -4.5802) -> (6.7394, -4.5218)
  line L2571 (6.7394, -4.5218) -> (6.7815, -4.4786)
  line L2572 (6.7815, -4.4786) -> (6.8439, -4.4182)
  line L2573 (6.8439, -4.4182) -> (6.8642, -4.3951)
  line L2574 (6.8642, -4.3951) -> (6.8807, -4.3732)
  line L2575 (6.8807, -4.3732) -> (6.8936, -4.3525)
  line L2576 (6.8936, -4.3525) -> (6.9028, -4.3333)
  line L2577 (6.9028, -4.3333) -> (6.9085, -4.3157)
  line L2578 (6.9085, -4.3157) -> (6.9107, -4.2998)
  line L2579 (6.9107, -4.2998) -> (6.9095, -4.2857)
  line L2580 (6.9095, -4.2857) -> (6.9049, -4.2737)
  line L2581 (6.9049, -4.2737) -> (6.8916, -4.2537)
  line L2582 (6.8916, -4.2537) -> (6.8144, -4.1359)
  line L2583 (6.8144, -4.1359) -> (6.7394, -4.0168)
  line L2584 (6.7394, -4.0168) -> (6.7267, -3.9963)
  line L2585 (6.7267, -3.9963) -> (6.7176, -3.9872)
  line L2586 (6.7176, -3.9872) -> (6.7053, -3.9802)
  line L2587 (6.7053, -3.9802) -> (6.69, -3.9756)
  line L2588 (6.69, -3.9756) -> (6.6716, -3.9735)
  line L2589 (6.6716, -3.9735) -> (6.6503, -3.9739)
  line L2590 (6.6503, -3.9739) -> (6.6262, -3.977)
  line L2591 (6.6262, -3.977) -> (6.5993, -3.9829)
  line L2592 (6.5993, -3.9829) -> (6.5698, -3.9918)
  line L2593 (6.5698, -3.9918) -> (6.489, -4.0235)
  line L2594 (6.489, -4.0235) -> (6.4323, -4.0438)
  line L2595 (6.4323, -4.0438) -> (6.3573, -4.0673)
  line L2596 (6.3573, -4.0673) -> (6.2708, -4.0904)
  line L2597 (6.2708, -4.0904) -> (6.1694, -4.1129)
  line L2598 (6.1694, -4.1129) -> (6.0547, -4.1335)
  line L2599 (6.0547, -4.1335) -> (5.9254, -4.1511)
  line L2600 (5.9254, -4.1511) -> (5.7809, -4.1647)
  line L2601 (5.7809, -4.1647) -> (5.7041, -4.1695)
  line L2602 (5.7041, -4.1695) -> (5.5599, -4.1742)
  arc A66 (5.3891, -3.8429) -> (5.5599, -4.1742) centre (13.25, 0) ccw
  line L2603 (5.3891, -3.8429) -> (5.4766, -3.7282)
  line L2604 (5.4766, -3.7282) -> (5.5251, -3.6684)
  line L2605 (5.5251, -3.6684) -> (5.6199, -3.5586)
  line L2606 (5.6199, -3.5586) -> (5.7093, -3.4635)
  line L2607 (5.7093, -3.4635) -> (5.7926, -3.3819)
  line L2608 (5.7926, -3.3819) -> (5.8698, -3.3125)
  line L2609 (5.8698, -3.3125) -> (5.9387, -3.2554)
  line L2610 (5.9387, -3.2554) -> (6.0013, -3.2079)
  line L2611 (6.0013, -3.2079) -> (6.0508, -3.1735)
  line L2612 (6.0508, -3.1735) -> (6.1235, -3.126)
  line L2613 (6.1235, -3.126) -> (6.1478, -3.1072)
  line L2614 (6.1478, -3.1072) -> (6.1682, -3.0887)
  line L2615 (6.1682, -3.0887) -> (6.1847, -3.0709)
  line L2616 (6.1847, -3.0709) -> (6.1974, -3.0538)
  line L2617 (6.1974, -3.0538) -> (6.2064, -3.0375)
  line L2618 (6.2064, -3.0375) -> (6.2115, -3.0223)
  line L2619 (6.2115, -3.0223) -> (6.213, -3.0083)
  line L2620 (6.213, -3.0083) -> (6.2108, -2.9957)
  line L2621 (6.2108, -2.9957) -> (6.2015, -2.9735)
  line L2622 (6.2015, -2.9735) -> (6.148, -2.8432)
  line L2623 (6.148, -2.8432) -> (6.0968, -2.712)
  line L2624 (6.0968, -2.712) -> (6.0882, -2.6895)
  line L2625 (6.0882, -2.6895) -> (6.0811, -2.6789)
  line L2626 (6.0811, -2.6789) -> (6.0703, -2.6697)
  line L2627 (6.0703, -2.6697) -> (6.0561, -2.6623)
  line L2628 (6.0561, -2.6623) -> (6.0385, -2.6567)
  line L2629 (6.0385, -2.6567) -> (6.0175, -2.6531)
  line L2630 (6.0175, -2.6531) -> (5.9932, -2.6516)
  line L2631 (5.9932, -2.6516) -> (5.9657, -2.6523)
  line L2632 (5.9657, -2.6523) -> (5.9351, -2.6554)
  line L2633 (5.9351, -2.6554) -> (5.8498, -2.6712)
  line L2634 (5.8498, -2.6712) -> (5.7902, -2.6805)
  line L2635 (5.7902, -2.6805) -> (5.7121, -2.6893)
  line L2636 (5.7121, -2.6893) -> (5.6228, -2.6956)
  line L2637 (5.6228, -2.6956) -> (5.519, -2.6986)
  line L2638 (5.519, -2.6986) -> (5.4024, -2.697)
  line L2639 (5.4024, -2.697) -> (5.2721, -2.6899)
  line L2640 (5.2721, -2.6899) -> (5.1277, -2.6759)
  line L2641 (5.1277, -2.6759) -> (5.0514, -2.666)
  line L2642 (5.0514, -2.666) -> (4.9089, -2.6434)
  arc A67 (4.8038, -2.2858) -> (4.9089, -2.6434) centre (13.25, 0) ccw
  line L2643 (4.8038, -2.2858) -> (4.9115, -2.1897)
  point P0 (0, 0)
  point P1 (4.8038, -2.2858)
  point P2 (4.9089, -2.6434)
  point P3 (5.3891, -3.8429)
  point P4 (5.5599, -4.1742)
  point P5 (6.2584, -5.2612)
  point P6 (6.4888, -5.5542)
  point P7 (7.3804, -6.4893)
  point P8 (7.6621, -6.7334)
  point P9 (8.7146, -7.4828)
  point P10 (9.0374, -7.6692)
  point P11 (10.2127, -8.2059)
  point P12 (10.5649, -8.3278)
  point P13 (11.8205, -8.6324)
  point P14 (12.1895, -8.6855)
  point P15 (13.4801, -8.747)
  point P16 (13.8524, -8.7292)
  point P17 (15.1313, -8.5454)
  point P18 (15.4935, -8.4575)
  point P19 (16.7145, -8.0349)
  point P20 (17.0536, -7.88)
  point P21 (18.1725, -7.234)
  point P22 (18.4762, -7.0178)
  point P23 (19.4526, -6.1717)
  point P24 (19.7098, -5.9019)
  point P25 (20.5085, -4.8863)
  point P26 (20.7101, -4.5727)
  point P27 (21.3021, -3.4243)
  point P28 (21.4406, -3.0783)
  point P29 (21.8047, -1.8386)
  point P30 (21.8752, -1.4726)
  point P31 (21.998, -0.1864)
  point P32 (21.998, 0.1864)
  point P33 (21.8752, 1.4726)
  point P34 (21.8047, 1.8386)
  point P35 (21.4406, 3.0783)
  point P36 (21.3021, 3.4243)
  point P37 (20.7101, 4.5727)
  point P38 (20.5085, 4.8863)
  point P39 (19.7098, 5.9019)
  point P40 (19.4526, 6.1717)
  point P41 (18.4762, 7.0178)
  point P42 (18.1725, 7.234)
  point P43 (17.0536, 7.88)
  point P44 (16.7145, 8.0349)
  point P45 (15.4935, 8.4575)
  point P46 (15.1313, 8.5454)
  point P47 (13.8524, 8.7292)
  point P48 (13.4801, 8.747)
  point P49 (12.1895, 8.6855)
  point P50 (11.8205, 8.6324)
  point P51 (10.5649, 8.3278)
  point P52 (10.2127, 8.2059)
  point P53 (9.0374, 7.6692)
  point P54 (8.7146, 7.4828)
  point P55 (7.6621, 6.7334)
  point P56 (7.3804, 6.4893)
  point P57 (6.4888, 5.5542)
  point P58 (6.2584, 5.2612)
  point P59 (5.5599, 4.1742)
  point P60 (5.3891, 3.8429)
  point P61 (4.9089, 2.6434)
  point P62 (4.8038, 2.2858)
  point P63 (4.5593, 1.0171)
  point P64 (4.5239, 0.646)
  point P65 (4.5239, -0.646)
  point P66 (4.5593, -1.0171)
  constraints: 5288 end point, 132 point on circle, 68 centre point
extrude "Extrusion1" add sketch "Sketch1" against normal blind 2
body "Solid1"
